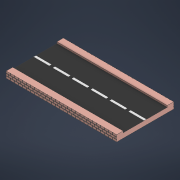
# Autodesk Inventor part: McCrea_most_cesta_walle
Saved by Autodesk Inventor 2022 (Build 260153000, 153)
## iProperties
Created: 2022-02-07
Part Number: McCrea_most_cesta_walle
Material: Generic
Document SubType Name: Modeling
Designer: MatusBarany
Density: 1 g/cm^3
Appearance: Default
Author: MatusBarany
Autodesk Inventor part; units mm, degrees
ref_plane "YZ Plane" through (0, 0, 0) normal (1, 0, 0) x (0, 1, 0)
ref_plane "XZ Plane" through (0, 0, 0) normal (0, 1, 0) x (-1, 0, 0)
ref_plane "XY Plane" through (0, 0, 0) normal (0, 0, 1) x (1, 0, 0)
sketch "Sketch1" plane through (0, 0, 0) normal (0, 0, 1) x (1, 0, 0)
  line L0 (-1804.1747, 240.1678) -> (1695.8253, 240.1678)
  line L1 (-1804.1747, 240.1678) -> (1695.8253, 240.1678)
  line L2 (1695.8253, 240.1678) -> (1695.8253, 390.1678)
  line L3 (1695.8253, 390.1678) -> (-1804.1747, 390.1678)
  line L4 (-1804.1747, 390.1678) -> (-1804.1747, 240.1678)
  line L5 (-1204.1747, 240.1678) -> (-1004.1747, 240.1678)
  line L6 (895.8253, 240.1678) -> (1095.8253, 240.1678)
  dimension "d2" = 150
  dimension "d9" = 3500
  constraints: 14 end point, 4 horizontal, 2 parallel, 2 point on line, 1 perpendicular
  measures "d2" distance of L1.end L2.end
  measures "d9" distance of L2.end L3.end
extrude "Extrusion1" add sketch "Sketch1" along normal blind 700
sketch "Sketch2" plane through (0, 0, 700) normal (0, 0, 1) x (1, 0, 0)
  line L0 (-1804.1747, 240.1678) -> (1695.8253, 240.1678) projected
  line L1 (1695.8253, 240.1678) -> (1695.8253, 390.1678) projected
  line L2 (1695.8253, 390.1678) -> (-1804.1747, 390.1678) projected
  line L3 (-1804.1747, 390.1678) -> (-1804.1747, 240.1678) projected
  line L4 (1695.8253, 390.1678) -> (-1804.1747, 390.1678) projected
  line L5 (-1804.1747, 390.1678) -> (1695.8253, 390.1678)
  line L6 (1695.8253, 390.1678) -> (1695.8253, 440.1678)
  line L7 (1695.8253, 440.1678) -> (-1804.1747, 440.1678)
  line L8 (-1804.1747, 440.1678) -> (-1804.1747, 390.1678)
  point P0 (0, 0)
  dimension "d12" = 50
  constraints: 8 end point, 2 parallel, 1 horizontal, 1 perpendicular
  measures "d12" distance of L5.end L6.end
extrude "Extrusion2" add sketch "Sketch2" along normal blind 200
mirror "Mirror1" about plane through (0, 0, 0) normal (0, 0, 1) of "Extrusion2", "Extrusion1"
sketch "Sketch3" plane through (-1804.1747, 390.1678, 700) normal (0, 1, 0) x (1, 0, 0)
  line L0 (0, 1400) -> (0, 0) projected
  line L1 (0, 740) -> (500, 740)
  line L2 (500, 740) -> (500, 660)
  line L3 (500, 660) -> (0, 660)
  line L4 (0, 660) -> (0, 740)
  line L5 (4200, 700) -> (-700, 700) projected
  point P0 (1804.1747, 700)
  dimension "d15" = 80
  dimension "d16" = 40
  dimension "d17" = 500
  constraints: 8 end point, 2 parallel, 1 horizontal, 1 perpendicular, 1 point on line
  measures "d15" distance of L1.end L2.end
  measures "d16" distance between parallel lines of L1 L5
  measures "d17" distance of L1.start L1.end
extrude "Extrusion3" add sketch "Sketch3" along normal blind 5
pattern_linear "Rectangular Pattern1" count 6 spacing 600 along (1, 0, 0) of "Extrusion3"
sketch "Sketch4" plane through (0, 0, 900) normal (0, 0, 1) x (1, 0, 0)
  line L0 (1695.8253, 240.1678) -> (1695.8253, 440.1678) projected
  line L1 (1695.8253, 440.1678) -> (-1804.1747, 440.1678) projected
  line L2 (-1804.1747, 440.1678) -> (-1804.1747, 240.1678) projected
  line L3 (-1804.1747, 240.1678) -> (1695.8253, 240.1678) projected
  line L4 (-1804.1747, 240.1678) -> (-1684.1747, 240.1678)
  line L5 (-1684.1747, 240.1678) -> (-1684.1747, 300.1678)
  line L6 (-1684.1747, 300.1678) -> (-1804.1747, 300.1678)
  line L7 (-1804.1747, 300.1678) -> (-1804.1747, 240.1678)
  line L8 (1695.8253, 440.1678) -> (-1804.1747, 440.1678) projected
  line L9 (-1804.1747, 380.1678) -> (-1684.1747, 380.1678)
  line L10 (-1684.1747, 380.1678) -> (-1684.1747, 440.1678)
  line L11 (-1684.1747, 440.1678) -> (-1804.1747, 440.1678)
  line L12 (-1804.1747, 440.1678) -> (-1804.1747, 380.1678)
  line L13 (-1804.1747, 310.1678) -> (-1744.1747, 310.1678)
  line L14 (-1744.1747, 310.1678) -> (-1744.1747, 370.1678)
  line L15 (-1744.1747, 370.1678) -> (-1804.1747, 370.1678)
  line L16 (-1804.1747, 370.1678) -> (-1804.1747, 310.1678)
  line L17 (-1734.1747, 310.1678) -> (-1614.1747, 310.1678)
  line L18 (-1614.1747, 310.1678) -> (-1614.1747, 370.1678)
  line L19 (-1614.1747, 370.1678) -> (-1734.1747, 370.1678)
  line L20 (-1734.1747, 370.1678) -> (-1734.1747, 310.1678)
  point P0 (0, 0)
  dimension "d23" = 200
  dimension "d24" = 60
  dimension "d25" = 120
  dimension "d26" = 60
  dimension "d27" = 120
  dimension "d28" = 60
  dimension "d29" = 10
  dimension "d30" = 60
  dimension "d31" = 120
  dimension "d32" = 60
  dimension "d33" = 10
  dimension "d34" = 10
  constraints: 32 end point, 8 parallel, 4 horizontal, 4 perpendicular, 3 point on line
  measures "d23" distance of L1.end L2.end
  measures "d24" distance of L4.end L5.end
  measures "d25" distance of L5.end L6.end
  measures "d26" distance of L9.end L10.end
  measures "d27" distance of L9.start L9.end
  measures "d28" distance of L13.end L14.end
  measures "d29" distance between parallel lines of L13 L6
  measures "d30" distance of L14.end L15.end
  measures "d31" distance of L18.end L19.end
  measures "d32" distance of L17.end L18.end
  measures "d33" distance between parallel lines of L14 L20
  measures "d34" distance between parallel lines of L9 L19
extrude "Extrusion4" add sketch "Sketch4" along normal blind 5 contours L3 L2 L6 L5 | L10 L9 L2 L1 | L2 L15 L14 L13 | L20 L19 L18 L17
pattern_linear "Rectangular Pattern2" count 26 spacing 130 along (1, 0, 0) of "Extrusion4"
sketch "Sketch5" plane through (0, 0, 900) normal (0, 0, 1) x (1, 0, 0)
  line L0 (1565.8253, 240.1678) -> (1695.8253, 240.1678) projected
  line L1 (1575.8253, 300.1678) -> (1695.8253, 300.1678)
  line L2 (1695.8253, 300.1678) -> (1695.8253, 240.1678)
  line L3 (1695.8253, 240.1678) -> (1575.8253, 240.1678)
  line L4 (1575.8253, 240.1678) -> (1575.8253, 300.1678)
  line L5 (1695.8253, 440.1678) -> (1575.8253, 440.1678)
  line L6 (1575.8253, 440.1678) -> (1575.8253, 380.1678)
  line L7 (1575.8253, 380.1678) -> (1695.8253, 380.1678)
  line L8 (1695.8253, 380.1678) -> (1695.8253, 440.1678)
  line L9 (1695.8253, 240.1678) -> (1695.8253, 440.1678) projected
  line L10 (1695.8253, 370.1678) -> (1645.8253, 370.1678)
  line L11 (1645.8253, 370.1678) -> (1645.8253, 310.1678)
  line L12 (1645.8253, 310.1678) -> (1695.8253, 310.1678)
  line L13 (1695.8253, 310.1678) -> (1695.8253, 370.1678)
  line L14 (1635.8253, 310.1678) -> (1635.8253, 370.1678) projected
  point P0 (0, 0)
  dimension "d40" = 120
  dimension "d41" = 60
  dimension "d42" = 120
  dimension "d43" = 60
  dimension "d44" = 10
  dimension "d45" = 50
  dimension "d46" = 10
  dimension "d49" = 60
  constraints: 24 end point, 6 parallel, 3 horizontal, 3 perpendicular, 1 point on line
  measures "d40" distance of L1.start L1.end
  measures "d41" distance of L3.end L1.start
  measures "d42" distance of L6.end L7.end
  measures "d43" distance of L5.end L6.end
  measures "d44" distance between parallel lines of L14 L11
  measures "d45" distance of L10.start L10.end
  measures "d46" distance between parallel lines of L1 L12
  measures "d49" distance of L10.end L11.end
extrude "Extrusion5" add sketch "Sketch5" along normal blind 5
mirror "Mirror2" about plane through (0, 0, 0) normal (0, 0, 1) of "Extrusion4", "Rectangular Pattern2", "Extrusion5"
equation "\"d42\" = d40"
equation "\"d43\" = d41"
body "Solid1"
